CXT (Autodesk Fusion 360 design; units mm, degrees)
Autodesk Fusion 360 part; units mm, degrees
note: some values were not read from the file. Set by a fixed rule: which sketch regions a step uses.
sketch "Sketch1" plane through (0, 0, 0) normal (1, 0, 0) x (0, 1, 0)
  line L0 (-85.8595, 38.3827) -> (-35.8595, 38.3827)
  line L1 (-35.8595, 38.3827) -> (-27.8595, 26.3827)
  line L2 (-27.8595, 26.3827) -> (-77.8595, 26.3827)
  line L3 (-77.8595, 26.3827) -> (-85.8595, 38.3827)
  line L4 (-39.8826, 38.3827) -> (-39.8826, 33.3827)
  line L5 (-39.8826, 33.3827) -> (-82.5261, 33.3827)
  line L6 (-85.8595, 38.3827) -> (-92.8595, 38.3827)
  line L7 (-92.8595, 38.3827) -> (-92.8595, 36.3827)
  line L8 (-92.8595, 36.3827) -> (-84.5261, 36.3827)
  line L9 (-77.8595, 26.3827) -> (-92.8595, 26.3827)
  line L10 (-92.8595, 26.3827) -> (-92.8595, 36.3827)
  line L11 (-92.8595, 26.3827) -> (-27.8595, 26.3827)
  line L12 (-27.8595, 26.3827) -> (-27.8595, 21.8827)
  line L13 (-27.8595, 21.8827) -> (-92.8595, 21.8827)
  line L14 (-92.8595, 21.8827) -> (-92.8595, 26.3827)
  line L15 (-40.8595, 26.3827) -> (-40.8595, 21.8827)
  line L16 (-73.8595, 26.3827) -> (-73.8595, 21.8827)
  line L17 (-40.8595, 25.1327) -> (-73.8595, 25.1327)
  line L18 (-73.8595, 23.1327) -> (-40.8595, 23.1327)
  line L19 (-43.8595, 25.1327) -> (-43.8595, 23.1327)
  line L20 (-70.8595, 25.1327) -> (-70.8595, 23.1327)
  line L21 (-64.8595, 26.3827) -> (-64.8595, 34.8827)
  line L22 (-64.8595, 34.8827) -> (-88.8595, 34.8827)
  line L23 (-27.8595, 26.3827) -> (-37.8595, 26.3827)
  line L24 (-27.8595, 21.8827) -> (-30.8595, 21.8827)
  line L25 (-30.8595, 21.8827) -> (-37.8595, 26.3827)
  line L26 (-27.8595, 21.8827) -> (-24.8595, 21.8827)
  line L27 (-24.8595, 21.8827) -> (-24.8595, 26.3827)
  line L28 (-24.8595, 26.3827) -> (-27.8595, 26.3827)
  line L29 (-27.8595, 26.3827) -> (-27.8595, 21.8827)
  line L30 (-92.8595, 35.3827) -> (-83.8595, 35.3827)
  dimension "d1" = 50
  dimension "d2" = 50
  dimension "d3" = 8
  dimension "d4" = 12
  dimension "d5" = 5
  dimension "d6" = 7
  dimension "d7" = 2
  dimension "d8" = 4.5
  dimension "d9" = 13
  dimension "d10" = 33
  dimension "d11" = 1.25
  dimension "d12" = 1.25
  dimension "d13" = 3
  dimension "d14" = 3
  dimension "d15" = 24
  dimension "d16" = 8.5
  dimension "d17" = 24
  dimension "d18" = 10
  dimension "d19" = 3
  dimension "d20" = 3
  dimension "d58" = 15
  dimension "d69" = 3
  constraint horizontal L0
  constraint parallel L0 L2
  constraint coincident L0 L4.start
  constraint perpendicular L0 L4
  constraint coincident L3 L5.end
  constraint perpendicular L4 L5
  constraint parallel L0 L6
  constraint perpendicular L6 L7
  constraint coincident L3 L8.end
  constraint perpendicular L7 L8
  constraint perpendicular L7 L9
  constraint perpendicular L8 L10
  constraint horizontal L11
  constraint vertical L12
  constraint horizontal L13
  constraint vertical L14
  constraint coincident L2 L15.start
  constraint coincident L13 L15.end
  constraint perpendicular L13 L15
  constraint coincident L11 L16.start
  constraint coincident L13 L16.end
  constraint perpendicular L13 L16
  constraint coincident L15 L17.start
  constraint coincident L16 L17.end
  constraint perpendicular L16 L17
  constraint coincident L16 L18.start
  constraint coincident L15 L18.end
  constraint perpendicular L15 L18
  constraint coincident L17 L19.start
  constraint coincident L18 L19.end
  constraint perpendicular L18 L19
  constraint coincident L17 L20.start
  constraint coincident L18 L20.end
  constraint perpendicular L18 L20
  constraint coincident L2 L21.start
  constraint perpendicular L2 L21
  constraint perpendicular L21 L22
  constraint perpendicular L12 L23
  constraint perpendicular L12 L24
  constraint horizontal L26
  constraint vertical L27
  constraint horizontal L28
  constraint vertical L29
  constraint coincident L1 L2.start
  constraint coincident L10 L30.start
  constraint coincident L3 L30.end
  constraint perpendicular L10 L30
  measures "d1" distance of L1.end L2.end
  measures "d2" distance of L0.start L0.end
  measures "d3" horizontal distance of L0.end L1.end
  measures "d4" vertical distance of L0.end L1.end
  measures "d5" distance of L4.start L4.end
  measures "d6" distance of L0.start L6.end
  measures "d7" distance of L6.end L7.end
  measures "d8" distance of L9.end L13.end
  measures "d9" distance of L12 L15
  measures "d10" distance of L15 L16
  measures "d11" distance of L2 L17
  measures "d12" distance of L13 L18
  measures "d13" distance of L15 L19
  measures "d14" distance of L16 L20
  measures "d15" distance of L15 L21
  measures "d16" distance of L21.start L21.end
  measures "d17" distance of L21.end L22.end
  measures "d18" distance of L1.end L23.end
  measures "d19" distance of L12.end L24.end
  measures "d20" distance of L12.end L26.end
  measures "d58" distance of L2.end L9.end
  measures "d69" distance of L6 L30
extrude "Extrude1" add sketch "Sketch1" along normal mid plane 30 contours L3 L9 L10 L11 L30 | L2 L3 L5 L11 L21 | L3 L5 L21 L22 makes body 1
extrude "Extrude2" add sketch "Sketch1" along normal mid plane 31 separate body contours L17 L18 L19 L20 makes body 2
extrude "Extrude3" add sketch "Sketch1" along normal mid plane 35 contours L2 L11 L15 L16 L17 | L13 L15 L16 L18 bodies 1 2
extrude "Extrude4" add sketch "Sketch1" along normal blind 4 from surface at 22 separate body contours L0 L3 L4 L5 L21 L22 | L3 L6 L7 L8 | L0 L1 L2 L4 L5 L11 L21 L23 | L3 L8 L10 L30 | L3 L9 L10 L11 L30 | L2 L11 L12 L13 L23 L24 L25 L29 | L12 L26 L27 L28 L29 | L2 L3 L5 L11 L21 | L3 L5 L21 L22 | L2 L11 L13 L15 L25 | L2 L11 L15 L16 L17 | L2 L9 L11 L13 L14 L16 | L15 L17 L18 L19 | L13 L15 L16 L18 | L16 L17 L18 L20 | L17 L18 L19 L20 makes body 3
extrude "Extrude5" add sketch "Sketch1" along normal blind 4 from surface at -26 separate body contours L0 L3 L4 L5 L21 L22 | L3 L6 L7 L8 | L0 L1 L2 L4 L5 L11 L21 L23 | L3 L8 L10 L30 | L3 L9 L10 L11 L30 | L2 L11 L12 L13 L23 L24 L25 L29 | L12 L26 L27 L28 L29 | L2 L3 L5 L11 L21 | L3 L5 L21 L22 | L2 L11 L13 L15 L25 | L2 L11 L15 L16 L17 | L2 L9 L11 L13 L14 L16 | L15 L17 L18 L19 | L13 L15 L16 L18 | L16 L17 L18 L20 | L17 L18 L19 L20 makes body 4
extrude "Extrude6" add sketch "Sketch1" along normal mid plane 27 separate body contours L2 L11 L12 L13 L23 L24 L25 L29 makes body 5
extrude "Extrude7" add sketch "Sketch1" against normal blind 2.5 from surface at 22 contours L0 L3 L4 L5 L21 L22 | L3 L6 L7 L8 | L3 L8 L10 L30 | L3 L5 L21 L22 bodies 3
extrude "Extrude8" add sketch "Sketch1" along normal blind 2.5 from surface at -22 contours L0 L3 L4 L5 L21 L22 | L3 L6 L7 L8 | L3 L8 L10 L30 | L3 L5 L21 L22 bodies 4
extrude "Extrude9" add sketch "Sketch1" along normal through all and the other way through all contours L3 L9 L10 L11 L30 | L2 L11 L12 L13 L23 L24 L25 L29 | L12 L26 L27 L28 L29 | L2 L11 L13 L15 L25 | L2 L11 L15 L16 L17 | L2 L9 L11 L13 L14 L16 | L15 L17 L18 L19 | L13 L15 L16 L18 | L16 L17 L18 L20 | L17 L18 L19 L20 bodies 3 4
combine "Combine1" operation cut target body 3 tool bodies 1 5
chamfer "Chamfer1" distance 2 angle 45 2 edges at (-20.75, -39.8826, 33.3827) (20.75, -39.8826, 33.3827) on bodies 3 4
sketch "Sketch2" plane through (0, 0, 21.8827) normal (0, 0, -1) x (1, 0, 0)
  line L0 (-13.5, 27.8595) -> (-13.5, 30.8595)
  line L1 (-13.5, 30.8595) -> (13.5, 30.8595)
  line L2 (13.5, 30.8595) -> (13.5, 27.8595)
  line L3 (13.5, 27.8595) -> (-13.5, 27.8595)
  line L4 (-17.5, 40.8595) -> (-17.5, 73.8595)
  line L5 (-17.5, 73.8595) -> (17.5, 73.8595)
  line L6 (17.5, 73.8595) -> (17.5, 40.8595)
  line L7 (17.5, 40.8595) -> (-17.5, 40.8595)
  line L8 (-26, 24.8595) -> (26, 24.8595)
  line L9 (26, 24.8595) -> (26, 92.8595)
  line L10 (26, 92.8595) -> (-26, 92.8595)
  line L11 (-26, 92.8595) -> (-26, 24.8595)
  line L12 (26, 24.8595) -> (33, 24.8595)
  line L13 (33, 24.8595) -> (33, 92.8595)
  line L14 (33, 92.8595) -> (26, 92.8595)
  line L15 (26, 92.8595) -> (26, 24.8595)
  line L16 (-26, 24.8595) -> (-33, 24.8595)
  line L17 (-33, 24.8595) -> (-33, 92.8595)
  line L18 (-33, 92.8595) -> (-26, 92.8595)
  line L19 (-26, 92.8595) -> (-26, 24.8595)
  line L20 (26, 24.8595) -> (-26, 24.8595)
  line L21 (-26, 24.8595) -> (-26, 92.8595)
  line L22 (-26, 92.8595) -> (26, 92.8595)
  line L23 (26, 92.8595) -> (26, 24.8595)
  circle A0 centre (29.5, 29.8595) radius 1.5
  circle A1 centre (-29.5, 29.8595) radius 1.5
  circle A2 centre (29.5, 58.8595) radius 1.5
  circle A3 centre (-29.5, 58.8595) radius 1.5
  circle A4 centre (29.5, 87.8595) radius 1.5
  circle A5 centre (-29.5, 87.8595) radius 1.5
  dimension "d43" = 7
  dimension "d44" = 7
  dimension "d45" = 3
  dimension "d46" = 5
  dimension "d47" = 3.5
  dimension "d50" = 59
  dimension "d51" = -58
  constraint horizontal L12
  constraint vertical L13
  constraint horizontal L14
  constraint vertical L15
  constraint coincident L8.end L9.start
  constraint horizontal L16
  constraint vertical L17
  constraint horizontal L18
  constraint vertical L19
  constraint coincident L8.start L11.end
  constraint horizontal L20
  constraint vertical L21
  constraint horizontal L22
  constraint vertical L23
  constraint coincident L10.end L11.start
  constraint coincident L18 L10.end
  constraint coincident L9.end L14
  measures "d43" distance of L8.end L12.end
  measures "d44" distance of L8.start L16.end
  measures "d45" diameter of A0
  measures "d46" distance of L12 A0.centre
  measures "d47" distance of L15 A0.centre
extrude "Extrude10" add sketch "Sketch2" along normal blind 3 contours L0 L1 L2 L3 | L8 L9 L10 L11 L15 L19 L20 L21 L22 L23 | L11 L16 L17 L18 L19 L21 | L9 L12 L13 L14 L15 L23 bodies 3
sketch "Sketch4" plane through (0, 0, 26.3827) normal (0, 0, 1) x (-1, 0, 0)
  line L0 (13.5, 37.8595) -> (13.5, 27.8595)
  line L1 (13.5, 27.8595) -> (-13.5, 27.8595)
  line L2 (-13.5, 27.8595) -> (-13.5, 37.8595)
  line L3 (-13.5, 37.8595) -> (13.5, 37.8595)
  line L4 (-15, 77.8595) -> (-22, 77.8595)
  line L5 (-22, 77.8595) -> (-22, 27.8595)
  line L6 (-22, 27.8595) -> (-26, 27.8595)
  line L7 (-26, 27.8595) -> (-26, 24.8595)
  line L8 (-26, 24.8595) -> (26, 24.8595)
  line L9 (26, 24.8595) -> (26, 27.8595)
  line L10 (26, 27.8595) -> (22, 27.8595)
  line L11 (22, 27.8595) -> (22, 77.8595)
  line L12 (22, 77.8595) -> (15, 77.8595)
  line L13 (15, 77.8595) -> (15, 92.8595)
  line L14 (15, 92.8595) -> (-15, 92.8595)
  line L15 (-15, 92.8595) -> (-15, 77.8595)
  line L16 (-17.5, 73.8595) -> (17.5, 73.8595)
  line L17 (17.5, 73.8595) -> (17.5, 40.8595)
  line L18 (17.5, 40.8595) -> (-17.5, 40.8595)
  line L19 (-17.5, 40.8595) -> (-17.5, 73.8595)
  line L20 (-15, 92.8595) -> (15, 92.8595)
  line L21 (15, 92.8595) -> (15, 69.346)
  line L22 (15, 69.346) -> (-15, 69.346)
  line L23 (-15, 69.346) -> (-15, 92.8595)
  line L24 (-15, 92.8595) -> (15, 92.8595)
  line L25 (15, 92.8595) -> (15, 87.8595)
  line L26 (15, 87.8595) -> (-15, 87.8595)
  line L27 (-15, 87.8595) -> (-15, 92.8595)
  line L28 (-17.5, 40.8595) -> (17.5, 40.8595)
  line L29 (17.5, 40.8595) -> (17.5, 73.8595)
  line L30 (17.5, 73.8595) -> (-17.5, 73.8595)
  line L31 (-17.5, 73.8595) -> (-17.5, 40.8595)
  line L32 (15.5, 70.8595) -> (15.5, 43.8595)
  line L33 (15.5, 43.8595) -> (-15.5, 43.8595)
  line L34 (-15.5, 43.8595) -> (-15.5, 70.8595)
  line L35 (-15.5, 70.8595) -> (15.5, 70.8595)
  dimension "d59" = 5
  constraint horizontal L20
  constraint vertical L21
  constraint horizontal L22
  constraint vertical L23
  constraint coincident L14.end L15.start
  constraint horizontal L24
  constraint vertical L25
  constraint horizontal L26
  constraint vertical L27
  constraint coincident L13 L25.end
  measures "d59" distance of L14.end L26.end
extrude "Extrude12" add sketch "Sketch4" along normal blind 9 contours L13 L14 L15 L20 L21 L23 L24 L25 L26 L27 bodies 3
extrude "Extrude13" cut sketch "Sketch4" against normal blind 20 contours L13 L15 L16 L21 L23 L26 L30 | L16 L21 L23 L30 L35 | L21 L22 L23 L35 bodies 3
ref_plane "WorkPlane2" through (0, -58.8595, 30.1327) normal (-1, 0, 0) x (0, -1, 0)
split "Split2" by plane through (0, -58.8595, 30.1327) normal (-1, 0, 0) bodies 3 makes body 6 at (-15.1723, -31.7849, 18.8827)
sketch "Sketch5" plane through (0, 0, 26.3827) normal (0, 0, 1) x (-1, 0, 0)
  line L0 (0, 37.8595) -> (0, 40.8595)
  line L1 (0, 40.8595) -> (-17.5, 40.8595)
  line L2 (-17.5, 40.8595) -> (-17.5, 73.8595)
  line L3 (-17.5, 73.8595) -> (-15, 73.8595)
  line L4 (-15, 73.8595) -> (-15, 77.8595)
  line L5 (-15, 77.8595) -> (-22, 77.8595)
  line L6 (-22, 77.8595) -> (-22, 27.8595)
  line L7 (-22, 27.8595) -> (-26, 27.8595)
  line L8 (-26, 27.8595) -> (-26, 24.8595)
  line L9 (-26, 24.8595) -> (0, 24.8595)
  line L10 (0, 24.8595) -> (0, 27.8595)
  line L11 (0, 27.8595) -> (-13.5, 27.8595)
  line L12 (-13.5, 27.8595) -> (-13.5, 37.8595)
  line L13 (-13.5, 37.8595) -> (0, 37.8595)
  line L14 (0, 40.8595) -> (0, 37.8595)
  line L15 (0, 37.8595) -> (13.5, 37.8595)
  line L16 (13.5, 37.8595) -> (13.5, 27.8595)
  line L17 (13.5, 27.8595) -> (0, 27.8595)
  line L18 (0, 27.8595) -> (0, 24.8595)
  line L19 (0, 24.8595) -> (26, 24.8595)
  line L20 (26, 24.8595) -> (26, 27.8595)
  line L21 (26, 27.8595) -> (22, 27.8595)
  line L22 (22, 27.8595) -> (22, 77.8595)
  line L23 (22, 77.8595) -> (15, 77.8595)
  line L24 (15, 77.8595) -> (15, 73.8595)
  line L25 (15, 73.8595) -> (17.5, 73.8595)
  line L26 (17.5, 73.8595) -> (17.5, 40.8595)
  line L27 (17.5, 40.8595) -> (0, 40.8595)
  line L28 (-13.5, 32.8595) -> (-26, 32.8595)
  line L29 (13.5, 32.8595) -> (26, 32.8595)
  line L30 (-26, 32.8595) -> (-26, 27.8595)
  line L31 (26, 32.8595) -> (26, 27.8595)
  constraint midpoint L12 L28.start
  constraint perpendicular L6 L28
  constraint midpoint L16 L29.start
  constraint perpendicular L22 L29
  constraint coincident L7.end L8.start
  constraint perpendicular L7 L30
  constraint coincident L20.end L21.start
  constraint perpendicular L21 L31
extrude "Extrude14" add sketch "Sketch5" along normal blind 1.5 contours L6 L7 L8 L9 L10 L11 L12 L18 L28 | L6 L7 L28 L30 bodies 3
extrude "Extrude15" add sketch "Sketch5" along normal blind 1.5 contours L10 L16 L17 L18 L19 L20 L21 L22 L29 | L21 L22 L29 L31 bodies 6
equation "d30 = -22 mm - 4 mm"
